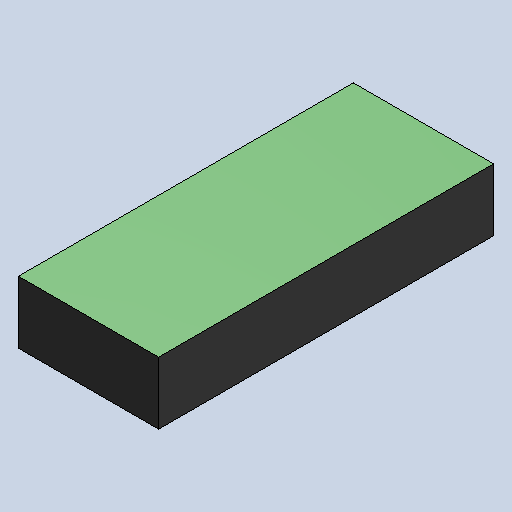
# Autodesk Inventor part: Talon 25A ESC
Saved by Autodesk Inventor 2023 (Build 270158000, 158)
## iProperties
Created: 2022-05-19
Part Number: Talon 25A ESC
Material: Generic
Document SubType Name: Modeling
Designer: Nathan Cai
Mass: 17.8602 g
Surface Area: 26.0541 cm^2
Volume: 6.494 cm^3
Density: 2.75026 g/cm^3
Appearance: Rubber - Black
Author: Nathan Cai
Autodesk Inventor part; units mm, degrees
ref_plane "YZ Plane" through (0, 0, 0) normal (1, 0, 0) x (0, 1, 0)
ref_plane "XZ Plane" through (0, 0, 0) normal (0, 1, 0) x (-1, 0, 0)
ref_plane "XY Plane" through (0, 0, 0) normal (0, 0, 1) x (1, 0, 0)
sketch "Sketch1" plane through (0, 0, 0) normal (0, 1, 0) x (-1, 0, 0)
  line L0 (-9.144, 21.844) -> (9.144, 21.844)
  line L1 (9.144, 21.844) -> (9.144, -21.844)
  line L2 (9.144, -21.844) -> (-9.144, -21.844)
  line L3 (-9.144, -21.844) -> (-9.144, 21.844)
  line L4 (-9.144, 21.844) -> (9.144, -21.844) construction
  line L5 (9.144, 21.844) -> (-9.144, -21.844) construction
  point P0 (0, 0)
  dimension "d0" = 18.288
  dimension "d1" = 43.688
  constraints: 12 end point, 2 midpoint, 2 parallel, 1 horizontal, 1 perpendicular
  measures "d0" distance of L1.end L2.end
  measures "d1" distance of L0.end L1.end
extrude "Extrusion1" add sketch "Sketch1" along normal blind 8.128
body "Solid1"
